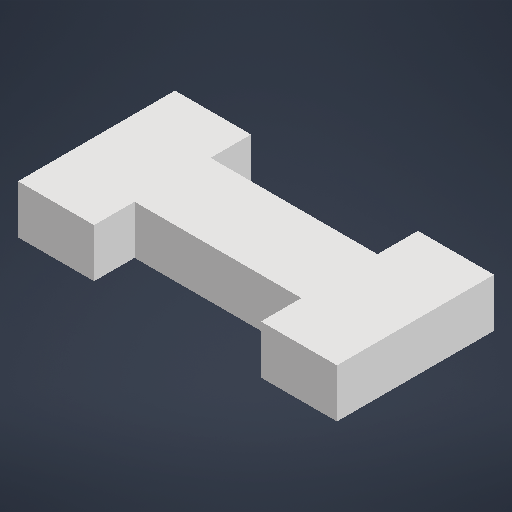
# Autodesk Inventor part: 3mmPin
Saved by Autodesk Inventor 2026 (Build 300175050, 175E)
## iProperties
Created: 2026-04-30
Part Number: 3mmPin
Material: Generic
Document SubType Name: Modeling
Designer: sniel
Density: 1 g/cm^3
Appearance: Default
Author: sniel
Autodesk Inventor part; units mm, degrees
ref_plane "YZ Plane" through (0, 0, 0) normal (1, 0, 0) x (0, 1, 0)
ref_plane "XZ Plane" through (0, 0, 0) normal (0, 1, 0) x (-1, 0, 0)
ref_plane "XY Plane" through (0, 0, 0) normal (0, 0, 1) x (1, 0, 0)
sketch "Sketch1" plane through (0, 0, 0) normal (0, 1, 0) x (-1, 0, 0)
  line L0 (15, -7.2) -> (15, 2.5)
  line L1 (15, 2.5) -> (10.3, 2.5)
  line L2 (10.3, 0) -> (10.3, 2.5)
  line L3 (10.3, 0) -> (0, 0)
  line L4 (0, 0) -> (0, 2.5)
  line L5 (0, 2.5) -> (-4.7, 2.5)
  line L6 (-4.7, 2.5) -> (-4.7, -7.2)
  line L7 (-4.7, -7.2) -> (0, -7.2)
  line L8 (0, -7.2) -> (0, -4.7)
  line L9 (0, -4.7) -> (10.3, -4.7)
  line L10 (10.3, -7.2) -> (10.3, -4.7)
  line L11 (15, -7.2) -> (10.3, -7.2)
  point P0 (0, 0)
  constraints: 24 end point
extrude "Extrusion1" add sketch "Sketch1" along normal blind 3
body "Solid1"
